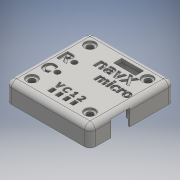
# Autodesk Inventor part: MyNavX_Mini_CoverV1.1
Saved by Autodesk Inventor 2016 (Build 200138000, 138)
## iProperties
Created: 2016-12-19
Part Number: MyNavX_Mini_CoverV1.1
Material: Generic
Document SubType Name: Modeling
Designer: Applefamily
Density: 1 g/cm^3
Appearance: Default
Author: Applefamily
Autodesk Inventor part; units mm, degrees
ref_plane "YZ Plane" through (0, 0, 0) normal (1, 0, 0) x (0, 1, 0)
ref_plane "XZ Plane" through (0, 0, 0) normal (0, 1, 0) x (-1, 0, 0)
ref_plane "XY Plane" through (0, 0, 0) normal (0, 0, 1) x (1, 0, 0)
sketch "Sketch1" plane through (0, 0, 0) normal (0, 0, 1) x (1, 0, 0)
  line L0 (-20.5, 23.5) -> (20.5, 23.5)
  line L1 (23.5, 20.5) -> (23.5, -20.5)
  line L2 (20.5, -23.5) -> (-20.5, -23.5)
  line L3 (-23.5, -20.5) -> (-23.5, 20.5)
  arc A0 (-20.5, 23.5) -> (-23.5, 20.5) centre (-20.5, 20.5) ccw
  arc A1 (23.5, 20.5) -> (20.5, 23.5) centre (20.5, 20.5) ccw
  arc A2 (20.5, -23.5) -> (23.5, -20.5) centre (20.5, -20.5) ccw
  arc A3 (-23.5, -20.5) -> (-20.5, -23.5) centre (-20.5, -20.5) ccw
  point P0 (0, 0)
  point P1 (-23.5, 23.5)
  point P2 (23.5, 23.5)
  point P3 (-23.5, -23.5)
  point P4 (-23.5, 0)
  point P5 (0, 23.5)
  dimension "d0" = 47
  dimension "d1" = 47
  dimension "d2" = 3
  constraints: 8 end point, 8 point on circle, 8 tangent, 6 point on line, 4 centre point, 3 equal radius, 2 midpoint, 2 parallel, 1 horizontal, 1 horizontal alignment, 1 perpendicular, 1 vertical alignment
  measures "d0" distance of point (-23.5, 23.5) point (23.5, 23.5)
  measures "d1" distance of point (-23.5, -23.5) point (-23.5, 23.5)
  measures "d2" radius of A0
extrude "Extrusion1" add sketch "Sketch1" along normal blind 2
sketch "Sketch2" plane through (0, 0, 2) normal (0, 0, 1) x (1, 0, 0)
  line L0 (-1, 18.75) -> (11.25, 18.75) projected
  line L1 (-1, 14.25) -> (-1, 18.75) projected
  line L2 (11.25, 14.25) -> (-1, 14.25) projected
  line L3 (11.25, 18.75) -> (11.25, 14.25) projected
  point P0 (0, 0)
extrude "Extrusion2" cut sketch "Sketch2" against normal blind 2
sketch "Sketch4" plane through (0, 0, 0) normal (0, 0, -1) x (-1, 0, 0)
  line L0 (20.5, 23.5) -> (-20.5, 23.5) projected
  arc A0 (-20.5, 23.5) -> (-23.5, 20.5) centre (-20.5, 20.5) ccw projected
  line L1 (-23.5, 20.5) -> (-23.5, -20.5) projected
  arc A1 (-23.5, -20.5) -> (-20.5, -23.5) centre (-20.5, -20.5) ccw projected
  line L2 (-20.5, -23.5) -> (20.5, -23.5) projected
  arc A2 (20.5, -23.5) -> (23.5, -20.5) centre (20.5, -20.5) ccw projected
  line L3 (23.5, -20.5) -> (23.5, 20.5) projected
  arc A3 (23.5, 20.5) -> (20.5, 23.5) centre (20.5, 20.5) ccw projected
  line L4 (20.5, -21.5) -> (-20.5, -21.5)
  arc A4 (-21.5, -20.5) -> (-20.5, -21.5) centre (-20.5, -20.5) ccw
  arc A5 (-20.5, 21.5) -> (-21.5, 20.5) centre (-20.5, 20.5) ccw
  line L5 (-20.5, 21.5) -> (20.5, 21.5)
  arc A6 (21.5, 20.5) -> (20.5, 21.5) centre (20.5, 20.5) ccw
  line L6 (21.5, 20.5) -> (21.5, -20.5)
  arc A7 (20.5, -21.5) -> (21.5, -20.5) centre (20.5, -20.5) ccw
  line L7 (-22.4, -1.25) -> (-21.5, -1.25) projected
  line L8 (-21.5, -11.75) -> (-22.4, -11.75) projected
  line L9 (-21.5, -11.75) -> (-23.5, -11.75)
  line L10 (-23.5, -1.25) -> (-21.5, -1.25)
  line L11 (-21.5, -20.5) -> (-21.5, -11.75)
  line L12 (-21.5, -1.25) -> (-21.5, 20.5)
  circle A8 centre (-16.25, -16.25) radius 1.75 projected
  circle A9 centre (16.25, 16.25) radius 1.75 projected
  circle A10 centre (-16.25, 16.25) radius 1.75 projected
  circle A11 centre (16.25, -16.25) radius 1.75 projected
  point P0 (0, 0)
  dimension "d8" = 2
  constraints: 14 end point, 8 point on circle, 4 centre point, 2 point on line, 1 collinear, 1 horizontal, 5 other
  measures "d8" distance between parallel lines of L2 L4
extrude "Extrusion3" add sketch "Sketch4" along normal blind 5.5 contours A3 L3 A2 L2 A1 L1 L9 L8 L11 A4 L4 A7 L6 A6 L5 A5 L12 L7 L10 A0 L0
sketch "Sketch5" plane through (0, 0, -5.5) normal (0, 0, -1) x (-1, 0, 0)
  line L0 (20.5, 23.5) -> (-20.5, 23.5) projected
  arc A0 (-20.5, 23.5) -> (-23.5, 20.5) centre (-20.5, 20.5) ccw projected
  line L1 (-23.5, 20.5) -> (-23.5, -1.25) projected
  line L2 (-23.5, -1.25) -> (-21.5, -1.25) projected
  line L3 (-21.5, -1.25) -> (-21.5, 20.5) projected
  arc A1 (-20.5, 21.5) -> (-21.5, 20.5) centre (-20.5, 20.5) ccw projected
  line L4 (-20.5, 21.5) -> (20.5, 21.5) projected
  arc A2 (21.5, 20.5) -> (20.5, 21.5) centre (20.5, 20.5) ccw projected
  line L5 (21.5, 20.5) -> (21.5, -20.5) projected
  arc A3 (20.5, -21.5) -> (21.5, -20.5) centre (20.5, -20.5) ccw projected
  line L6 (20.5, -21.5) -> (-20.5, -21.5) projected
  arc A4 (-21.5, -20.5) -> (-20.5, -21.5) centre (-20.5, -20.5) ccw projected
  line L7 (-21.5, -20.5) -> (-21.5, -11.75) projected
  line L8 (-21.5, -11.75) -> (-23.5, -11.75) projected
  line L9 (-23.5, -11.75) -> (-23.5, -20.5) projected
  arc A5 (-23.5, -20.5) -> (-20.5, -23.5) centre (-20.5, -20.5) ccw projected
  line L10 (-20.5, -23.5) -> (20.5, -23.5) projected
  arc A6 (20.5, -23.5) -> (23.5, -20.5) centre (20.5, -20.5) ccw projected
  line L11 (23.5, -20.5) -> (23.5, 20.5) projected
  arc A7 (23.5, 20.5) -> (20.5, 23.5) centre (20.5, 20.5) ccw projected
  line L12 (-22.6, -1.25) -> (-22.6, 20.5)
  arc A8 (-20.5, 22.6) -> (-22.6, 20.5) centre (-20.5, 20.5) ccw
  line L13 (-20.5, 22.6) -> (20.5, 22.6)
  arc A9 (22.6, 20.5) -> (20.5, 22.6) centre (20.5, 20.5) ccw
  line L14 (22.6, 20.5) -> (22.6, -20.5)
  arc A10 (20.5, -22.6) -> (22.6, -20.5) centre (20.5, -20.5) ccw
  line L15 (20.5, -22.6) -> (-20.5, -22.6)
  arc A11 (-22.6, -20.5) -> (-20.5, -22.6) centre (-20.5, -20.5) ccw
  line L16 (-22.6, -20.5) -> (-22.6, -11.75)
  arc A12 (-22.4, -20.5) -> (-20.5, -22.4) centre (-20.5, -20.5) ccw
  line L17 (-20.5, -22.4) -> (20.5, -22.4)
  arc A13 (20.5, -22.4) -> (22.4, -20.5) centre (20.5, -20.5) ccw
  line L18 (22.4, -20.5) -> (22.4, 20.5)
  arc A14 (22.4, 20.5) -> (20.5, 22.4) centre (20.5, 20.5) ccw
  line L19 (20.5, 22.4) -> (-20.5, 22.4)
  arc A15 (-20.5, 22.4) -> (-22.4, 20.5) centre (-20.5, 20.5) ccw
  point P0 (0, 0)
  dimension "d11" = 0.9
  constraints: 16 end point, 16 point on circle, 8 centre point, 2 point on line, 12 other
  measures "d11" distance between parallel lines of L1 L12
extrude "Extrusion4" add sketch "Sketch5" along normal blind 3.5 contours A7 L11 A6 L10 A5 L9 L8 L16 A11 L15 A10 L14 A9 L13 A8 L12 L2 L1 A0 L0
sketch "Sketch6" plane through (0, 0, 0) normal (0, 0, -1) x (-1, 0, 0)
  circle A0 centre (-16.25, 16.25) radius 1.75
  circle A1 centre (16.25, 16.25) radius 1.75
  circle A2 centre (16.25, -16.25) radius 1.75
  circle A3 centre (-16.25, -16.25) radius 1.75
  circle A4 centre (-16.25, 16.25) radius 3
  circle A5 centre (16.25, 16.25) radius 3
  circle A6 centre (-16.25, -16.25) radius 3
  circle A7 centre (16.25, -16.25) radius 3
  point P0 (0, 0)
  dimension "d14" = 6
  dimension "d15" = 6
  dimension "d16" = 6
  dimension "d17" = 6
  dimension "d52" = 3.5
  dimension "d53" = 3.5
  dimension "d54" = 3.5
  dimension "d55" = 3.5
  constraints: 8 centre point, 4 coincident
  measures "d14" diameter of A4
  measures "d15" diameter of A5
  measures "d16" diameter of A6
  measures "d17" diameter of A7
  measures "d52" diameter of A2
  measures "d53" diameter of A3
  measures "d54" diameter of A0
  measures "d55" diameter of A1
extrude "Extrusion5" cut sketch "Sketch6" against normal blind 2 contours A0 | A1 | A2 | A3
extrude "Extrusion6" add sketch "Sketch6" along normal blind 8.9
sketch "Sketch7" plane through (0, 0, 2) normal (0, 0, 1) x (1, 0, 0)
  circle A0 centre (-12.25, 3.5) radius 1.5
  circle A1 centre (-12.25, -6) radius 1.5
  line L0 (-23.5, 20.5) -> (-23.5, -20.5) projected
  line L1 (20.5, 23.5) -> (-20.5, 23.5) projected
  line L2 (-6, -14.7) -> (-4, -14.7)
  line L3 (-4, -14.7) -> (-4, -17.7)
  line L4 (-4, -17.7) -> (-6, -17.7)
  line L5 (-6, -17.7) -> (-6, -14.7)
  line L6 (-20.5, -23.5) -> (20.5, -23.5) projected
  line L7 (-1.9, -14.7) -> (0.1, -14.7)
  line L8 (0.1, -14.7) -> (0.1, -17.7)
  line L9 (0.1, -17.7) -> (-1.9, -17.7)
  line L10 (-1.9, -17.7) -> (-1.9, -14.7)
  line L11 (2.2, -14.7) -> (4.2, -14.7)
  line L12 (4.2, -14.7) -> (4.2, -17.7)
  line L13 (4.2, -17.7) -> (2.2, -17.7)
  line L14 (2.2, -17.7) -> (2.2, -14.7)
  line L15 (6.3, -14.7) -> (8.3, -14.7)
  line L16 (8.3, -14.7) -> (8.3, -17.7)
  line L17 (8.3, -17.7) -> (6.3, -17.7)
  line L18 (6.3, -17.7) -> (6.3, -14.7)
  point P0 (0, 0)
  dimension "d22" = 11.25
  dimension "d23" = 3
  dimension "d24" = 3
  dimension "d25" = 9.5
  dimension "d26" = 20
  dimension "d27" = 5.8
  dimension "d28" = 3
  dimension "d29" = 2
  dimension "d32" = 4.1
  dimension "d37" = 14.3
  dimension "d38" = 17.5
  constraints: 32 end point, 2 centre point, 2 horizontal, 2 parallel, 1 perpendicular, 1 vertical alignment, 24 other
  measures "d22" distance from line of L0 A0.centre
  measures "d23" diameter of A0
  measures "d24" diameter of A1
  measures "d25" distance of A1.centre A0.centre
  measures "d26" distance from line of L1 A0.centre
  measures "d27" distance between parallel lines of L6 L4
  measures "d28" distance of L4.end L2.start
  measures "d29" distance of L2.start L2.end
  measures "d32" distance of L2.start L7.start
  measures "d37" distance between parallel lines of L16 L5
  measures "d38" distance between parallel lines of L0 L5
extrude "Extrusion7" cut sketch "Sketch7" against normal blind 2
sketch "Sketch8" plane through (0, 0, 2) normal (0, 0, 1) x (1, 0, 0)
  circle A0 centre (-16.25, -16.25) radius 1.75 projected
  circle A1 centre (-16.25, -16.25) radius 3
  circle A2 centre (16.1833, -16.25) radius 3
  circle A3 centre (16.1833, 16.0277) radius 3
  circle A4 centre (-16.25, 16.25) radius 1.75 projected
  circle A5 centre (-16.25, 16.25) radius 3
  point P0 (0, 0)
  dimension "d41" = 6
  dimension "d42" = 6
  dimension "d43" = 6
  dimension "d44" = 6
  constraints: 4 centre point, 2 coincident
  measures "d41" diameter of A1
  measures "d42" diameter of A2
  measures "d43" diameter of A3
  measures "d44" diameter of A5
extrude "Extrusion8" cut sketch "Sketch8" against normal blind 1
fillet "Fillet1" radius 3 8 edges at (-22.6213, -22.6213, 2) (0, -23.5, 2) (22.6213, -22.6213, 2) (23.5, 0, 2) (22.6213, 22.6213, 2) (0, 23.5, 2) (-22.6213, 22.6213, 2) (-23.5, 0, 2)
sketch "Sketch10" plane through (0, 0, 2) normal (0, 0, 1) x (1, 0, 0)
  line L0 (-6.1205, 13.3229) -> (19.7835, 13.3229) construction
  line L1 (19.7835, 13.3229) -> (19.7835, 3.9258) construction
  line L2 (19.7835, 3.9258) -> (-6.1205, 3.9258) construction
  line L3 (-6.1205, 3.9258) -> (-6.1205, 13.3229) construction
  line L4 (0.8037, 5.9041) -> (24.7294, 5.9041) construction
  line L5 (24.7294, 5.9041) -> (24.7294, -5.5332) construction
  line L6 (24.7294, -5.5332) -> (0.8037, -5.5332) construction
  line L7 (0.8037, -5.5332) -> (0.8037, 5.9041) construction
  line L8 (-19.8939, -2.8374) -> (-14.0915, -2.8374) construction
  line L9 (-14.0915, -2.8374) -> (-14.0915, -7.1095) construction
  line L10 (-14.0915, -7.1095) -> (-19.8939, -7.1095) construction
  line L11 (-19.8939, -7.1095) -> (-19.8939, -2.8374) construction
  line L12 (-20.0214, 6.8545) -> (-14.9204, 6.8545) construction
  line L13 (-14.9204, 6.8545) -> (-14.9204, 2.4549) construction
  line L14 (-14.9204, 2.4549) -> (-20.0214, 2.4549) construction
  line L15 (-20.0214, 2.4549) -> (-20.0214, 6.8545) construction
  line L16 (-6.8776, -10.0544) -> (-3.8115, -10.0544) construction
  line L17 (-3.8115, -10.0544) -> (-3.8115, -13.7018) construction
  line L18 (-3.8115, -13.7018) -> (-6.8776, -13.7018) construction
  line L19 (-6.8776, -13.7018) -> (-6.8776, -10.0544) construction
  line L20 (-2.6855, -10.0544) -> (0.528, -10.0544) construction
  line L21 (0.528, -10.0544) -> (0.528, -13.6905) construction
  line L22 (0.528, -13.6905) -> (-2.6855, -13.6905) construction
  line L23 (-2.6855, -13.6905) -> (-2.6855, -10.0544) construction
  line L24 (1.703, -10.1199) -> (4.7691, -10.1199) construction
  line L25 (4.7691, -10.1199) -> (4.7691, -13.6284) construction
  line L26 (4.7691, -13.6284) -> (1.703, -13.6284) construction
  line L27 (1.703, -13.6284) -> (1.703, -10.1199) construction
  line L28 (5.8296, -10.1854) -> (8.8956, -10.1854) construction
  line L29 (8.8956, -10.1854) -> (8.8956, -13.7534) construction
  line L30 (8.8956, -13.7534) -> (5.8296, -13.7534) construction
  line L31 (5.8296, -13.7534) -> (5.8296, -10.1854) construction
  line L32 (-13.7533, 0.7545) -> (-15.6169, 0.7545)
  line L33 (-15.6169, 0.7545) -> (-17.3125, 2.9938)
  line L34 (-17.3125, 2.9938) -> (-17.8661, 2.9938)
  line L35 (-17.8661, 2.9938) -> (-17.8661, 0.7545)
  line L36 (-17.8661, 0.7545) -> (-19.3887, 0.7545)
  line L37 (-19.3887, 0.7545) -> (-19.3887, 6.8545)
  line L38 (-19.3887, 6.8545) -> (-16.9368, 6.8545)
  spline S0 degree 2 poles (-16.9368, 6.8545) (-16.4276, 6.8545) (-15.6763, 6.7259) (-15.3549, 6.5282) knots 0 0 0 1 2 2 2
  spline S1 degree 2 poles (-15.3549, 6.5282) (-15.0287, 6.3206) (-14.6431, 5.673) (-14.6431, 5.1787) knots 0 0 0 1 2 2 2
  spline S2 degree 2 poles (-14.6431, 5.1787) (-14.6431, 4.4817) (-15.2758, 3.6067) (-15.8048, 3.3497) knots 0 0 0 1 2 2 2
  line L39 (-15.8048, 3.3497) -> (-13.7533, 0.7545)
  spline S3 degree 2 poles (-16.2151, 4.9859) (-16.2151, 5.2182) (-16.393, 5.5494) (-16.5957, 5.6384) knots 0 0 0 1 2 2 2
  spline S4 degree 2 poles (-16.5957, 5.6384) (-16.7391, 5.6977) (-17.09, 5.7323) (-17.352, 5.7323) knots 0 0 0 1 2 2 2
  line L40 (-17.352, 5.7323) -> (-17.8661, 5.7323)
  line L41 (-17.8661, 5.7323) -> (-17.8661, 4.0912)
  line L42 (-17.8661, 4.0912) -> (-17.4262, 4.0912)
  spline S5 degree 2 poles (-17.4262, 4.0912) (-17.1098, 4.0912) (-16.66, 4.1703) (-16.5067, 4.2938) knots 0 0 0 1 2 2 2
  spline S6 degree 2 poles (-16.5067, 4.2938) (-16.3584, 4.4125) (-16.2151, 4.7288) (-16.2151, 4.9859) knots 0 0 0 1 2 2 2
  spline S7 degree 2 poles (-16.6313, -9.1747) (-18.0055, -9.1747) (-19.617, -7.5138) (-19.617, -6.011) knots 0 0 0 1 2 2 2
  spline S8 degree 2 poles (-19.617, -6.011) (-19.617, -4.5626) (-18.0006, -2.8374) (-16.6264, -2.8374) knots 0 0 0 1 2 2 2
  spline S9 degree 2 poles (-16.6264, -2.8374) (-16.2655, -2.8374) (-15.6822, -2.9215) (-15.4153, -2.9907) knots 0 0 0 1 2 2 2
  spline S10 degree 2 poles (-15.4153, -2.9907) (-15.2076, -3.0549) (-14.7183, -3.2675) (-14.565, -3.3466) knots 0 0 0 1 2 2 2
  line L43 (-14.565, -3.3466) -> (-14.565, -4.7999)
  line L44 (-14.565, -4.7999) -> (-14.7183, -4.7999)
  spline S11 degree 2 poles (-14.7183, -4.7999) (-14.832, -4.701) (-15.1681, -4.4242) (-15.3807, -4.2957) knots 0 0 0 1 2 2 2
  spline S12 degree 2 poles (-15.3807, -4.2957) (-15.5932, -4.1622) (-16.1024, -3.9793) (-16.3841, -3.9793) knots 0 0 0 1 2 2 2
  spline S13 degree 2 poles (-16.3841, -3.9793) (-16.7153, -3.9793) (-17.264, -4.1869) (-17.5162, -4.4489) knots 0 0 0 1 2 2 2
  spline S14 degree 2 poles (-17.5162, -4.4489) (-17.7435, -4.6813) (-18.0352, -5.4771) (-18.0352, -6.016) knots 0 0 0 1 2 2 2
  spline S15 degree 2 poles (-18.0352, -6.016) (-18.0352, -6.5844) (-17.7337, -7.3605) (-17.4865, -7.5978) knots 0 0 0 1 2 2 2
  spline S16 degree 2 poles (-17.4865, -7.5978) (-17.2492, -7.8301) (-16.6659, -8.0328) (-16.3743, -8.0328) knots 0 0 0 1 2 2 2
  spline S17 degree 2 poles (-16.3743, -8.0328) (-16.0727, -8.0328) (-15.524, -7.8301) (-15.3362, -7.7066) knots 0 0 0 1 2 2 2
  spline S18 degree 2 poles (-15.3362, -7.7066) (-15.1286, -7.583) (-14.8171, -7.321) (-14.7034, -7.2172) knots 0 0 0 1 2 2 2
  line L45 (-14.7034, -7.2172) -> (-14.565, -7.2172)
  line L46 (-14.565, -7.2172) -> (-14.565, -8.6507)
  spline S19 degree 2 poles (-14.565, -8.6507) (-14.7331, -8.7298) (-15.173, -8.9275) (-15.4103, -8.9967) knots 0 0 0 1 2 2 2
  spline S20 degree 2 poles (-15.4103, -8.9967) (-15.697, -9.0857) (-16.1963, -9.1747) (-16.6313, -9.1747) knots 0 0 0 1 2 2 2
  line L47 (-3.5931, -10.0544) -> (-4.7957, -13.5544)
  line L48 (-4.7957, -13.5544) -> (-5.7119, -13.5544)
  line L49 (-5.7119, -13.5544) -> (-6.9144, -10.0544)
  line L50 (-6.9144, -10.0544) -> (-6.004, -10.0544)
  line L51 (-6.004, -10.0544) -> (-5.241, -12.4283)
  line L52 (-5.241, -12.4283) -> (-4.4809, -10.0544)
  line L53 (-4.4809, -10.0544) -> (-3.5931, -10.0544)
  spline S21 degree 2 poles (-0.8136, -13.6905) (-1.6021, -13.6905) (-2.5267, -12.7375) (-2.5267, -11.8753) knots 0 0 0 1 2 2 2
  spline S22 degree 2 poles (-2.5267, -11.8753) (-2.5267, -11.0442) (-1.5992, -10.0544) (-0.8107, -10.0544) knots 0 0 0 1 2 2 2
  spline S23 degree 2 poles (-0.8107, -10.0544) (-0.6037, -10.0544) (-0.269, -10.1026) (-0.1158, -10.1423) knots 0 0 0 1 2 2 2
  spline S24 degree 2 poles (-0.1158, -10.1423) (0.0033, -10.1791) (0.2841, -10.3011) (0.372, -10.3465) knots 0 0 0 1 2 2 2
  line L54 (0.372, -10.3465) -> (0.372, -11.1804)
  line L55 (0.372, -11.1804) -> (0.2841, -11.1804)
  spline S25 degree 2 poles (0.2841, -11.1804) (0.2188, -11.1236) (0.026, -10.9648) (-0.096, -10.8911) knots 0 0 0 1 2 2 2
  spline S26 degree 2 poles (-0.096, -10.8911) (-0.2179, -10.8145) (-0.5101, -10.7095) (-0.6718, -10.7095) knots 0 0 0 1 2 2 2
  spline S27 degree 2 poles (-0.6718, -10.7095) (-0.8618, -10.7095) (-1.1766, -10.8287) (-1.3213, -10.979) knots 0 0 0 1 2 2 2
  spline S28 degree 2 poles (-1.3213, -10.979) (-1.4517, -11.1123) (-1.6191, -11.5689) (-1.6191, -11.8781) knots 0 0 0 1 2 2 2
  spline S29 degree 2 poles (-1.6191, -11.8781) (-1.6191, -12.2043) (-1.4461, -12.6496) (-1.3042, -12.7857) knots 0 0 0 1 2 2 2
  spline S30 degree 2 poles (-1.3042, -12.7857) (-1.1681, -12.919) (-0.8334, -13.0353) (-0.6661, -13.0353) knots 0 0 0 1 2 2 2
  spline S31 degree 2 poles (-0.6661, -13.0353) (-0.4931, -13.0353) (-0.1782, -12.919) (-0.0705, -12.8481) knots 0 0 0 1 2 2 2
  spline S32 degree 2 poles (-0.0705, -12.8481) (0.0487, -12.7772) (0.2274, -12.6269) (0.2926, -12.5673) knots 0 0 0 1 2 2 2
  line L56 (0.2926, -12.5673) -> (0.372, -12.5673)
  line L57 (0.372, -12.5673) -> (0.372, -13.3898)
  spline S33 degree 2 poles (0.372, -13.3898) (0.2756, -13.4352) (0.0231, -13.5487) (-0.113, -13.5884) knots 0 0 0 1 2 2 2
  spline S34 degree 2 poles (-0.113, -13.5884) (-0.2775, -13.6394) (-0.564, -13.6905) (-0.8136, -13.6905) knots 0 0 0 1 2 2 2
  line L58 (4.4741, -13.6284) -> (2.1625, -13.6284)
  line L59 (2.1625, -13.6284) -> (2.1625, -13.0186)
  line L60 (2.1625, -13.0186) -> (2.8999, -13.0186)
  line L61 (2.8999, -13.0186) -> (2.8999, -11.1664)
  line L62 (2.8999, -11.1664) -> (2.1625, -11.1664)
  line L63 (2.1625, -11.1664) -> (2.1625, -10.5964)
  spline S35 degree 2 poles (2.1625, -10.5964) (2.3242, -10.5964) (2.6447, -10.5538) (2.7411, -10.5084) knots 0 0 0 1 2 2 2
  spline S36 degree 2 poles (2.7411, -10.5084) (2.8517, -10.4517) (2.9765, -10.2617) (2.9879, -10.1199) knots 0 0 0 1 2 2 2
  line L64 (2.9879, -10.1199) -> (3.7537, -10.1199)
  line L65 (3.7537, -10.1199) -> (3.7537, -13.0186)
  line L66 (3.7537, -13.0186) -> (4.4741, -13.0186)
  line L67 (4.4741, -13.0186) -> (4.4741, -13.6284)
  line L68 (8.7566, -13.7534) -> (6.1841, -13.7534)
  line L69 (6.1841, -13.7534) -> (6.1841, -13.1833)
  spline S37 degree 2 poles (6.1841, -13.1833) (6.5103, -12.9224) (7.0322, -12.4629) (7.2279, -12.2559) knots 0 0 0 1 2 2 2
  spline S38 degree 2 poles (7.2279, -12.2559) (7.486, -11.9864) (7.7157, -11.5751) (7.7157, -11.3596) knots 0 0 0 1 2 2 2
  spline S39 degree 2 poles (7.7157, -11.3596) (7.7157, -11.1157) (7.4236, -10.8547) (7.1626, -10.8547) knots 0 0 0 1 2 2 2
  spline S40 degree 2 poles (7.1626, -10.8547) (7.0293, -10.8547) (6.7911, -10.92) (6.6691, -10.971) knots 0 0 0 1 2 2 2
  spline S41 degree 2 poles (6.6691, -10.971) (6.55, -11.0249) (6.3798, -11.1384) (6.3373, -11.1667) knots 0 0 0 1 2 2 2
  line L70 (6.3373, -11.1667) -> (6.2692, -11.1667)
  line L71 (6.2692, -11.1667) -> (6.2692, -10.4037)
  spline S42 degree 2 poles (6.2692, -10.4037) (6.4167, -10.3328) (7.0463, -10.1854) (7.3385, -10.1854) knots 0 0 0 1 2 2 2
  spline S43 degree 2 poles (7.3385, -10.1854) (7.9625, -10.1854) (8.6035, -10.7413) (8.6035, -11.2433) knots 0 0 0 1 2 2 2
  spline S44 degree 2 poles (8.6035, -11.2433) (8.6035, -11.5525) (8.3113, -12.1481) (7.9738, -12.4884) knots 0 0 0 1 2 2 2
  spline S45 degree 2 poles (7.9738, -12.4884) (7.7611, -12.6983) (7.3612, -13.0245) (7.2732, -13.0926) knots 0 0 0 1 2 2 2
  line L72 (7.2732, -13.0926) -> (8.7566, -13.0926)
  line L73 (8.7566, -13.0926) -> (8.7566, -13.7534)
  line L74 (5.7551, 0.6772) -> (5.7551, 2.5613)
  spline S46 degree 2 poles (5.7551, 2.5613) (5.7551, 2.8409) (5.7348, 3.2218) (5.6862, 3.3434) knots 0 0 0 1 2 2 2
  spline S47 degree 2 poles (5.6862, 3.3434) (5.6335, 3.4649) (5.4228, 3.5743) (5.2324, 3.5743) knots 0 0 0 1 2 2 2
  spline S48 degree 2 poles (5.2324, 3.5743) (5.0987, 3.5743) (4.8394, 3.4568) (4.6854, 3.3474) knots 0 0 0 1 2 2 2
  line L75 (4.6854, 3.3474) -> (4.6854, 0.6772)
  line L76 (4.6854, 0.6772) -> (3.5022, 0.6772)
  line L77 (3.5022, 0.6772) -> (3.5022, 2.5613)
  spline S49 degree 2 poles (3.5022, 2.5613) (3.5022, 2.8369) (3.4779, 3.2218) (3.4293, 3.3434) knots 0 0 0 1 2 2 2
  spline S50 degree 2 poles (3.4293, 3.3434) (3.3766, 3.4649) (3.1659, 3.5743) (2.9755, 3.5743) knots 0 0 0 1 2 2 2
  spline S51 degree 2 poles (2.9755, 3.5743) (2.8337, 3.5743) (2.5541, 3.4406) (2.4244, 3.3474) knots 0 0 0 1 2 2 2
  line L78 (2.4244, 3.3474) -> (2.4244, 0.6772)
  line L79 (2.4244, 0.6772) -> (1.2494, 0.6772)
  line L80 (1.2494, 0.6772) -> (1.2494, 4.4495)
  line L81 (1.2494, 4.4495) -> (2.4244, 4.4495)
  line L82 (2.4244, 4.4495) -> (2.4244, 4.0322)
  spline S52 degree 2 poles (2.4244, 4.0322) (2.7121, 4.2753) (3.2267, 4.5508) (3.5468, 4.5508) knots 0 0 0 1 2 2 2
  spline S53 degree 2 poles (3.5468, 4.5508) (3.8912, 4.5508) (4.418, 4.2226) (4.5557, 3.8944) knots 0 0 0 1 2 2 2
  spline S54 degree 2 poles (4.5557, 3.8944) (4.892, 4.2105) (5.4917, 4.5508) (5.7997, 4.5508) knots 0 0 0 1 2 2 2
  spline S55 degree 2 poles (5.7997, 4.5508) (6.063, 4.5508) (6.4804, 4.3847) (6.6222, 4.2145) knots 0 0 0 1 2 2 2
  spline S56 degree 2 poles (6.6222, 4.2145) (6.7802, 4.0322) (6.9382, 3.5338) (6.9382, 3.1327) knots 0 0 0 1 2 2 2
  line L83 (6.9382, 3.1327) -> (6.9382, 0.6772)
  line L84 (6.9382, 0.6772) -> (5.7551, 0.6772)
  line L85 (8.9844, 0.6772) -> (7.8094, 0.6772)
  line L86 (7.8094, 0.6772) -> (7.8094, 4.4495)
  line L87 (7.8094, 4.4495) -> (8.9844, 4.4495)
  line L88 (8.9844, 4.4495) -> (8.9844, 0.6772)
  line L89 (9.0209, 4.9884) -> (7.777, 4.9884)
  line L90 (7.777, 4.9884) -> (7.777, 5.9041)
  line L91 (7.777, 5.9041) -> (9.0209, 5.9041)
  line L92 (9.0209, 5.9041) -> (9.0209, 4.9884)
  spline S57 degree 2 poles (11.7316, 0.5759) (11.2656, 0.5759) (10.4917, 0.8109) (10.204, 1.0541) knots 0 0 0 1 2 2 2
  spline S58 degree 2 poles (10.204, 1.0541) (9.9244, 1.3012) (9.6084, 2.0427) (9.6084, 2.5451) knots 0 0 0 1 2 2 2
  spline S59 degree 2 poles (9.6084, 2.5451) (9.6084, 3.0881) (9.9488, 3.8458) (10.2445, 4.0889) knots 0 0 0 1 2 2 2
  spline S60 degree 2 poles (10.2445, 4.0889) (10.5241, 4.3239) (11.2859, 4.5508) (11.6992, 4.5508) knots 0 0 0 1 2 2 2
  spline S61 degree 2 poles (11.6992, 4.5508) (12.0112, 4.5508) (12.6351, 4.4049) (12.9512, 4.2469) knots 0 0 0 1 2 2 2
  line L93 (12.9512, 4.2469) -> (12.9512, 3.2421)
  line L94 (12.9512, 3.2421) -> (12.8013, 3.2421)
  spline S62 degree 2 poles (12.8013, 3.2421) (12.7283, 3.3109) (12.5257, 3.473) (12.4042, 3.5378) knots 0 0 0 1 2 2 2
  spline S63 degree 2 poles (12.4042, 3.5378) (12.2745, 3.6108) (11.9544, 3.708) (11.7559, 3.708) knots 0 0 0 1 2 2 2
  spline S64 degree 2 poles (11.7559, 3.708) (11.3061, 3.708) (10.8118, 3.08) (10.8118, 2.5451) knots 0 0 0 1 2 2 2
  spline S65 degree 2 poles (10.8118, 2.5451) (10.8118, 1.9779) (11.3386, 1.4187) (11.7762, 1.4187) knots 0 0 0 1 2 2 2
  spline S66 degree 2 poles (11.7762, 1.4187) (11.999, 1.4187) (12.3313, 1.52) (12.4528, 1.593) knots 0 0 0 1 2 2 2
  spline S67 degree 2 poles (12.4528, 1.593) (12.5703, 1.6618) (12.7405, 1.8158) (12.8013, 1.8766) knots 0 0 0 1 2 2 2
  line L95 (12.8013, 1.8766) -> (12.9512, 1.8766)
  line L96 (12.9512, 1.8766) -> (12.9512, 0.8677)
  spline S68 degree 2 poles (12.9512, 0.8677) (12.8499, 0.8231) (12.5865, 0.7096) (12.4488, 0.6732) knots 0 0 0 1 2 2 2
  spline S69 degree 2 poles (12.4488, 0.6732) (12.2786, 0.6246) (11.9787, 0.5759) (11.7316, 0.5759) knots 0 0 0 1 2 2 2
  line L97 (16.0428, 3.3353) -> (15.9455, 3.3353)
  spline S70 degree 2 poles (15.9455, 3.3353) (15.8766, 3.3596) (15.6214, 3.3839) (15.4674, 3.3839) knots 0 0 0 1 2 2 2
  spline S71 degree 2 poles (15.4674, 3.3839) (15.2851, 3.3839) (14.8758, 3.2745) (14.6854, 3.2015) knots 0 0 0 1 2 2 2
  line L98 (14.6854, 3.2015) -> (14.6854, 0.6772)
  line L99 (14.6854, 0.6772) -> (13.5103, 0.6772)
  line L100 (13.5103, 0.6772) -> (13.5103, 4.4495)
  line L101 (13.5103, 4.4495) -> (14.6854, 4.4495)
  line L102 (14.6854, 4.4495) -> (14.6854, 3.9066)
  spline S72 degree 2 poles (14.6854, 3.9066) (14.7664, 3.9795) (15.0501, 4.2064) (15.1676, 4.2753) knots 0 0 0 1 2 2 2
  spline S73 degree 2 poles (15.1676, 4.2753) (15.2972, 4.3523) (15.6376, 4.4617) (15.7875, 4.4617) knots 0 0 0 1 2 2 2
  spline S74 degree 2 poles (15.7875, 4.4617) (15.8442, 4.4617) (15.986, 4.4536) (16.0428, 4.4495) knots 0 0 0 1 2 2 2
  line L103 (16.0428, 4.4495) -> (16.0428, 3.3353)
  spline S75 degree 2 poles (20.1108, 2.5613) (20.1108, 1.6294) (19.0938, 0.5597) (18.1659, 0.5597) knots 0 0 0 1 2 2 2
  spline S76 degree 2 poles (18.1659, 0.5597) (17.2421, 0.5597) (16.217, 1.6294) (16.217, 2.5613) knots 0 0 0 1 2 2 2
  spline S77 degree 2 poles (16.217, 2.5613) (16.217, 3.5014) (17.2421, 4.567) (18.1659, 4.567) knots 0 0 0 1 2 2 2
  spline S78 degree 2 poles (18.1659, 4.567) (19.0898, 4.567) (20.1108, 3.4973) (20.1108, 2.5613) knots 0 0 0 1 2 2 2
  spline S79 degree 2 poles (18.9074, 2.5532) (18.9074, 2.8896) (18.798, 3.3393) (18.7008, 3.473) knots 0 0 0 1 2 2 2
  spline S80 degree 2 poles (18.7008, 3.473) (18.5954, 3.6148) (18.3321, 3.7242) (18.1659, 3.7242) knots 0 0 0 1 2 2 2
  spline S81 degree 2 poles (18.1659, 3.7242) (18.0039, 3.7242) (17.7486, 3.627) (17.6433, 3.4892) knots 0 0 0 1 2 2 2
  spline S82 degree 2 poles (17.6433, 3.4892) (17.542, 3.3596) (17.4204, 2.9017) (17.4204, 2.5532) knots 0 0 0 1 2 2 2
  spline S83 degree 2 poles (17.4204, 2.5532) (17.4204, 2.2088) (17.5339, 1.7834) (17.627, 1.6537) knots 0 0 0 1 2 2 2
  spline S84 degree 2 poles (17.627, 1.6537) (17.7202, 1.5241) (18.0039, 1.4025) (18.174, 1.4025) knots 0 0 0 1 2 2 2
  spline S85 degree 2 poles (18.174, 1.4025) (18.3159, 1.4025) (18.6076, 1.5241) (18.6967, 1.6456) knots 0 0 0 1 2 2 2
  spline S86 degree 2 poles (18.6967, 1.6456) (18.798, 1.7874) (18.9074, 2.1967) (18.9074, 2.5532) knots 0 0 0 1 2 2 2
  line L104 (-1.3458, 7.3229) -> (-2.7656, 7.3229)
  line L105 (-2.7656, 7.3229) -> (-2.7656, 9.5644)
  spline S87 degree 2 poles (-2.7656, 9.5644) (-2.7656, 9.8416) (-2.8093, 10.3862) (-2.8677, 10.5126) knots 0 0 0 1 2 2 2
  spline S88 degree 2 poles (-2.8677, 10.5126) (-2.9406, 10.6682) (-3.2129, 10.7994) (-3.4463, 10.7994) knots 0 0 0 1 2 2 2
  spline S89 degree 2 poles (-3.4463, 10.7994) (-3.6165, 10.7994) (-3.9714, 10.6682) (-4.1708, 10.5272) knots 0 0 0 1 2 2 2
  line L106 (-4.1708, 10.5272) -> (-4.1708, 7.3229)
  line L107 (-4.1708, 7.3229) -> (-5.5808, 7.3229)
  line L108 (-5.5808, 7.3229) -> (-5.5808, 11.8497)
  line L109 (-5.5808, 11.8497) -> (-4.1708, 11.8497)
  line L110 (-4.1708, 11.8497) -> (-4.1708, 11.3489)
  spline S90 degree 2 poles (-4.1708, 11.3489) (-3.8255, 11.6406) (-3.1691, 11.9712) (-2.7704, 11.9712) knots 0 0 0 1 2 2 2
  spline S91 degree 2 poles (-2.7704, 11.9712) (-2.08, 11.9712) (-1.3458, 11.096) (-1.3458, 10.2695) knots 0 0 0 1 2 2 2
  line L111 (-1.3458, 10.2695) -> (-1.3458, 7.3229)
  spline S92 degree 2 poles (2.1939, 7.8043) (2.048, 7.6828) (1.8195, 7.4883) (1.625, 7.391) knots 0 0 0 1 2 2 2
  spline S93 degree 2 poles (1.625, 7.391) (1.4354, 7.2986) (1.0756, 7.2014) (0.7547, 7.2014) knots 0 0 0 1 2 2 2
  spline S94 degree 2 poles (0.7547, 7.2014) (0.1518, 7.2014) (-0.6408, 8.0085) (-0.6408, 8.6212) knots 0 0 0 1 2 2 2
  spline S95 degree 2 poles (-0.6408, 8.6212) (-0.6408, 9.122) (-0.2372, 9.7443) (0.142, 9.9242) knots 0 0 0 1 2 2 2
  spline S96 degree 2 poles (0.142, 9.9242) (0.5262, 10.109) (1.591, 10.2549) (2.2036, 10.2938) knots 0 0 0 1 2 2 2
  line L112 (2.2036, 10.2938) -> (2.2036, 10.3181)
  spline S97 degree 2 poles (2.2036, 10.3181) (2.2036, 10.6925) (1.6493, 10.9793) (1.095, 10.9793) knots 0 0 0 1 2 2 2
  spline S98 degree 2 poles (1.095, 10.9793) (0.8471, 10.9793) (0.1761, 10.7994) (-0.14, 10.6584) knots 0 0 0 1 2 2 2
  line L113 (-0.14, 10.6584) -> (-0.2615, 10.6584)
  line L114 (-0.2615, 10.6584) -> (-0.2615, 11.7524)
  spline S99 degree 2 poles (-0.2615, 11.7524) (-0.0524, 11.8108) (0.8811, 11.9761) (1.3576, 11.9761) knots 0 0 0 1 2 2 2
  spline S100 degree 2 poles (1.3576, 11.9761) (2.5245, 11.9761) (3.5942, 11.1982) (3.5942, 10.4007) knots 0 0 0 1 2 2 2
  line L115 (3.5942, 10.4007) -> (3.5942, 7.3229)
  line L116 (3.5942, 7.3229) -> (2.1939, 7.3229)
  line L117 (2.1939, 7.3229) -> (2.1939, 7.8043)
  line L118 (2.1939, 8.5045) -> (2.1939, 9.4429)
  spline S101 degree 2 poles (2.1939, 9.4429) (1.8341, 9.4088) (1.3916, 9.3554) (1.1777, 9.2776) knots 0 0 0 1 2 2 2
  spline S102 degree 2 poles (1.1777, 9.2776) (0.9881, 9.2144) (0.7839, 8.9518) (0.7839, 8.7379) knots 0 0 0 1 2 2 2
  spline S103 degree 2 poles (0.7839, 8.7379) (0.7839, 8.4218) (1.1291, 8.1836) (1.4646, 8.1836) knots 0 0 0 1 2 2 2
  spline S104 degree 2 poles (1.4646, 8.1836) (1.6493, 8.1836) (2.0383, 8.3537) (2.1939, 8.5045) knots 0 0 0 1 2 2 2
  line L119 (8.8746, 11.8497) -> (7.2506, 7.3229)
  line L120 (7.2506, 7.3229) -> (5.7093, 7.3229)
  line L121 (5.7093, 7.3229) -> (4.0999, 11.8497)
  line L122 (4.0999, 11.8497) -> (5.5829, 11.8497)
  line L123 (5.5829, 11.8497) -> (6.5067, 8.8594)
  line L124 (6.5067, 8.8594) -> (7.4208, 11.8497)
  line L125 (7.4208, 11.8497) -> (8.8746, 11.8497)
  line L126 (14.5732, 7.3229) -> (12.8325, 7.3229)
  line L127 (12.8325, 7.3229) -> (11.6753, 9.2338)
  line L128 (11.6753, 9.2338) -> (10.4937, 7.3229)
  line L129 (10.4937, 7.3229) -> (8.826, 7.3229)
  line L130 (8.826, 7.3229) -> (10.7758, 10.3424)
  line L131 (10.7758, 10.3424) -> (8.9038, 13.3229)
  line L132 (8.9038, 13.3229) -> (10.6445, 13.3229)
  line L133 (10.6445, 13.3229) -> (11.7288, 11.5093)
  line L134 (11.7288, 11.5093) -> (12.8422, 13.3229)
  line L135 (12.8422, 13.3229) -> (14.51, 13.3229)
  line L136 (14.51, 13.3229) -> (12.6283, 10.4056)
  line L137 (12.6283, 10.4056) -> (14.5732, 7.3229)
  point P0 (0, 0)
  dimension "d0" = 47
  dimension "d1" = 47
  dimension "d2" = 3
  constraints: 16 other
emboss "Emboss2" sketch "Sketch10" operation cut depth 1 direction (0, 0, -1)
chamfer "Chamfer1" distance 0.25 angle 45 4 edges at (-19.25, 16.25, 1) (13.1833, 16.0277, 1) (-19.25, -16.25, 1) (13.1833, -16.25, 1)
equation "\"d53\" = d52"
equation "\"d54\" = d52"
equation "\"d55\" = d52"
equation "\"d24\" = d23"
equation "\"d41\" = d44"
equation "\"d42\" = d44"
equation "\"d43\" = d44"
equation "\"d1\" = d0"
body "Solid1"
